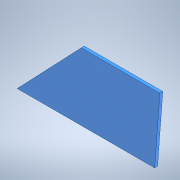
# Autodesk Inventor part: Tail Fin
Saved by Autodesk Inventor 2020 (Build 240168000, 168)
## iProperties
Created: 2022-11-08
Part Number: Tail Fin
Material: FibreGlass
Document SubType Name: Modeling
Designer: Hp
Density: 1500 g/cm^3
Appearance: Cyan
Author: Hp
Autodesk Inventor part; units mm, degrees
ref_plane "YZ Plane" through (0, 0, 0) normal (1, 0, 0) x (0, 1, 0)
ref_plane "XZ Plane" through (0, 0, 0) normal (0, 1, 0) x (-1, 0, 0)
ref_plane "XY Plane" through (0, 0, 0) normal (0, 0, 1) x (1, 0, 0)
sketch "Sketch1" plane through (0, 0, 0) normal (0, 0, 1) x (1, 0, 0)
  line L0 (0, 0) -> (-140, 0)
  line L1 (-140, 0) -> (-74.693, 68.5791)
  line L2 (-74.693, 68.5791) -> (5.307, 68.5791)
  line L3 (5.307, 68.5791) -> (0, 0)
  dimension "d0" = 140
  dimension "d1" = 94.7
  dimension "d2" = 46.4
  dimension "d3" = 80
  constraints: 8 end point, 1 horizontal, 1 parallel
  measures "d0" distance of L0.start L0.end
  measures "d1" distance of L0.end L1.end
  measures "d2" angle of L0 L1
  measures "d3" distance of L1.end L2.end
extrude "Extrusion1" add sketch "Sketch1" along normal blind 3
body "Solid1"
